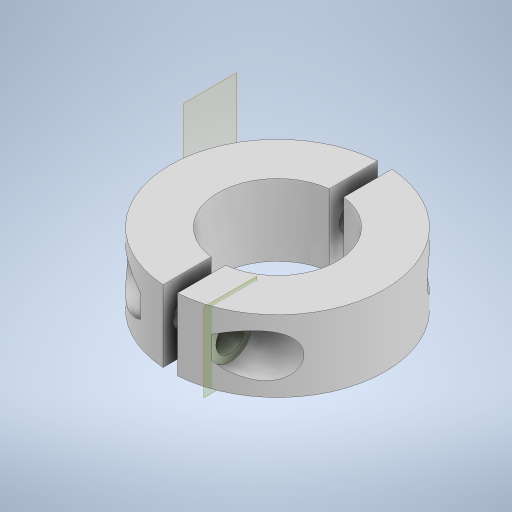
# Autodesk Inventor part: collar
Saved by Autodesk Inventor 2023 (Build 270158000, 158)
## iProperties
Created: 2022-11-03
Part Number: collar
Material: Generic
Document SubType Name: Modeling
Designer: neera
Density: 1 g/cm^3
Appearance: Default
Author: neera
Autodesk Inventor part; units mm, degrees
ref_plane "YZ Plane" through (0, 0, 0) normal (1, 0, 0) x (0, 1, 0)
ref_plane "XZ Plane" through (0, 0, 0) normal (0, 1, 0) x (-1, 0, 0)
ref_plane "XY Plane" through (0, 0, 0) normal (0, 0, 1) x (1, 0, 0)
sketch "Sketch1" plane through (0, 0, 0) normal (0, 1, 0) x (-1, 0, 0)
  circle A0 centre (0, 0) radius 4.15
  circle A1 centre (0, 0) radius 7.5
  dimension "d0" = 8.3
  dimension "d1" = 15
  constraints: 2 centre point, 2 coincident
  measures "d0" diameter of A0
  measures "d1" diameter of A1
extrude "Extrusion1" add sketch "Sketch1" along normal blind 5
sketch "Sketch2" plane through (0, 5, 0) normal (0, 1, 0) x (1, 0, 0)
  line L0 (-0.5, -8.297) -> (0.5, -8.297)
  line L1 (0.5, -8.297) -> (0.5, 8.8641)
  line L2 (0.5, 8.8641) -> (-0.5, 8.8641)
  line L3 (-0.5, 8.8641) -> (-0.5, -8.297)
  point P0 (0, 0)
  dimension "d4" = 1
  dimension "d5" = 0.5
  constraints: 8 end point, 2 parallel, 1 horizontal, 1 perpendicular
  measures "d4" distance of L2.end L1.end
  measures "d5" distance from line of point (0, 0) L3
extrude "Extrusion2" cut sketch "Sketch2" against normal blind 5
sketch "Sketch3" plane through (-0.5, 5, -4.1198) normal (1, 0, 0) x (0, 0, -1)
  circle A0 centre (1.6815, -2.5) radius 1
  line L0 (3.3635, -5) -> (3.3635, 0) projected
  line L1 (3.3635, -5) -> (-11.6031, -5) projected
  circle A1 centre (-9.9211, -2.5) radius 1
  line L2 (3.3635, 0) -> (-11.6031, 0) projected
  line L3 (-11.6031, 0) -> (-11.6031, -5) projected
  point P0 (-4.1198, -5)
  dimension "d8" = 2
  dimension "d9" = 1.682
  dimension "d10" = 2.5
  dimension "d11" = 2
  dimension "d12" = 2.5
  dimension "d13" = 1.682
  constraints: 2 centre point
  measures "d8" diameter of A0
  measures "d9" distance from line of L0 A0.centre
  measures "d10" distance from line of A0.centre L1
  measures "d11" diameter of A1
  measures "d12" distance from line of L2 A1.centre
  measures "d13" distance from line of L3 A1.centre
extrude "Extrusion3" cut sketch "Sketch3" along normal mid plane 20 contours A0 | A1
ref_plane "Work Plane1" through (-10.5, 5, -4.1198) normal (1, 0, 0) x (0, 0, -1)
sketch "Sketch4" plane through (-10.5, 5, -4.1198) normal (1, 0, 0) x (0, 0, -1)
  circle A0 centre (1.6815, -2.5) radius 1.5
  circle A1 centre (-9.9211, -2.5) radius 1.5
  circle A2 centre (-9.9211, -2.5) radius 1 projected
  circle A3 centre (1.6815, -2.5) radius 1 projected
  point P0 (-4.1198, -5)
  dimension "d17" = 3
  dimension "d18" = 3
  constraints: 2 centre point, 2 concentric
  measures "d17" diameter of A0
  measures "d18" diameter of A1
extrude "Extrusion4" cut sketch "Sketch4" along normal blind 8 contours A0 | A1 | A2 | A3
ref_plane "Work Plane2" through (2.5, 5, 4.1198) normal (-1, 0, 0) x (0, 0, 1)
sketch "Sketch6" plane through (2.5, 5, 4.1198) normal (-1, 0, 0) x (0, 0, 1)
  arc A0 (2.9513, -1.7014) -> (2.9513, -3.2986) centre (1.6815, -2.5) ccw projected
  circle A1 centre (1.6815, -2.5) radius 1.5
  circle A2 centre (-9.9211, -2.5) radius 1 projected
  circle A3 centre (-9.9211, -2.5) radius 1.5
  point P0 (-4.1198, -5)
  point P1 (2.9513, -3.2986)
  dimension "d31" = 3
  dimension "d32" = 3
  constraints: 2 centre point, 2 coincident
  measures "d31" diameter of A1
  measures "d32" diameter of A3
extrude "Extrusion6" cut sketch "Sketch6" against normal blind 10 contours A1 A0 | A2 | A3
body "Solid1"
